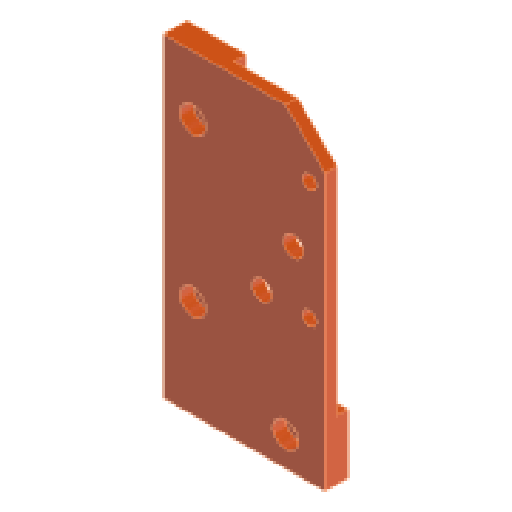
# Autodesk Inventor part: Alpha Idler Top
Saved by Autodesk Inventor 2023.2 (Build 272271000, 271)
## iProperties
Created: 2023-02-03
Part Number: Alpha Idler Top
Material: ABS Plastic
Document SubType Name: Modeling
Designer: remop
Density: 1.06 g/cm^3
Appearance: Smooth - Light Orange
Author: remop
Autodesk Inventor part; units mm, degrees
ref_plane "YZ Plane" through (0, 0, 0) normal (1, 0, 0) x (0, 1, 0)
ref_plane "XZ Plane" through (0, 0, 0) normal (0, 1, 0) x (-1, 0, 0)
ref_plane "XY Plane" through (0, 0, 0) normal (0, 0, 1) x (1, 0, 0)
sketch "Sketch1" plane through (0, 0, 0) normal (0, 0, 1) x (1, 0, 0)
  line L0 (-4, 11.7077) -> (6, 1.7077) projected
  line L1 (-4, 11.7077) -> (-5, 11.7077) projected
  arc A0 (-5, 11.7077) -> (-6, 10.7077) centre (-5, 10.7077) ccw projected
  line L2 (-6, 10.7077) -> (-6, -9.2784) projected
  arc A1 (-6, -9.2784) -> (-4.6842, -10.2272) centre (-5, -9.2784) ccw projected
  arc A2 (3.1184, -11.5061) -> (-4.6842, -10.2272) centre (-2, -18.2923) ccw projected
  arc A3 (3.1184, -11.5061) -> (3.7205, -11.7077) centre (3.7205, -10.7077) ccw projected
  line L3 (3.7205, -11.7077) -> (5, -11.7077) projected
  arc A4 (5, -11.7077) -> (6, -10.7077) centre (5, -10.7077) ccw projected
  line L4 (6, -10.7077) -> (6, 1.7077) projected
  arc A5 (5, -36.8923) -> (6, -35.8923) centre (5, -35.8923) ccw projected
  line L5 (6, -35.8923) -> (6, -27.7923) projected
  arc A6 (6, -27.7923) -> (5, -26.7923) centre (5, -27.7923) ccw projected
  line L6 (5, -26.7923) -> (-1.4303, -26.7923) projected
  arc A7 (-1.4303, -26.7923) -> (-2.3324, -28.2239) centre (-1.4303, -27.7923) ccw projected
  arc A8 (-2.2902, -35.4712) -> (-2.3324, -28.2239) centre (-10, -31.8923) ccw projected
  arc A9 (-2.2902, -35.4712) -> (-1.3832, -36.8923) centre (-1.3832, -35.8923) ccw projected
  line L7 (-1.3832, -36.8923) -> (5, -36.8923) projected
  line L8 (6, -53.1923) -> (6, -35.8923) projected
  line L9 (6, -27.7923) -> (6, -10.7077) projected
  line L10 (-5, 11.7077) -> (-20, 11.7077) projected
  line L11 (-20, 11.7077) -> (-35, 11.7077) projected
  line L12 (6, -68.1923) -> (6, -53.1923) projected
  line L13 (-35, 306.8077) -> (-35, -53.1923) projected
  line L14 (-35, -68.1923) -> (-35, -53.1923) projected
  line L15 (-20, -68.1923) -> (-35, -68.1923) projected
  line L16 (480, -68.1923) -> (-20, -68.1923) projected
  circle A10 centre (2, -2.1923) radius 1.4 projected
  circle A11 centre (2, -32.1923) radius 1.4 projected
  circle A12 centre (2, -2.1923) radius 1.75
  circle A13 centre (2, -32.1923) radius 1.75
  circle A14 centre (-10, -31.9923) radius 2.5 projected
  circle A15 centre (-2, -18.3923) radius 2.5 projected
  point P0 (0, 0)
  dimension "d18" = 3.5
  constraints: 2 centre point, 2 coincident, 1 equal radius
  measures "d18" diameter of A12
extrude "Extrusion1" add sketch "Sketch1" along normal blind 3 contours L0 L4 A4 L3 A3 A2 A1 L2 A0 L1 | A0 L2 A1 A2 A3 L3 A4 L9 A6 L6 A7 A8 A9 L7 A5 L8 L12 L16 L15 L14 L13 L11 L10 | L5 A5 L7 A9 A8 A7 L6 A6
sketch "Sketch2" plane through (0, 0, 0) normal (0, 0, -1) x (-1, 0, 0)
  line L0 (-6, -68.1923) -> (-6, 1.7077) projected
  line L1 (35, -68.1923) -> (-6, -68.1923) projected
  line L2 (35, 11.7077) -> (35, -68.1923) projected
  line L3 (4, 11.7077) -> (35, 11.7077) projected
  line L4 (-6, 1.7077) -> (4, 11.7077) projected
  line L5 (20, 11.7077) -> (20, -53.1923)
  line L6 (20, -53.1923) -> (-6, -53.1923)
  line L7 (-6, -68.1923) -> (-6, 1.7077) projected
  point P0 (0, 0)
  point P1 (7, -53.1923)
  dimension "d2" = 15
  dimension "d3" = 15
  constraints: 4 end point, 2 perpendicular, 2 point on line, 1 midpoint
  measures "d2" distance between parallel lines of L2 L5
  measures "d3" distance from line of L1 point (7, -53.192)
extrude "Extrusion2" add sketch "Sketch2" along normal blind 3 contours L0 L6 L5 L3 L2 L1
sketch "Sketch3" plane through (0, 0, 3) normal (0, 0, 1) x (1, 0, 0)
  line L0 (6, -68.1923) -> (6, 1.7077) projected
  line L1 (6, 1.7077) -> (-4, 11.7077) projected
  line L2 (-4, 11.7077) -> (-35, 11.7077) projected
  line L3 (-35, 11.7077) -> (-35, -68.1923) projected
  line L4 (-35, -68.1923) -> (6, -68.1923) projected
  circle A0 centre (2, -2.2923) radius 1.4 projected
  circle A1 centre (2, -32.2923) radius 1.4 projected
  point P0 (0, 0)
  point P1 (-27.5, -3.2923)
  point P2 (-27.5, -43.2923)
  point P3 (-4, -60.6923)
  dimension "d6" = 7.5
  dimension "d7" = 10
  dimension "d8" = 7.5
  dimension "d9" = 15
  dimension "d10" = 40
  constraints: 2 coincident, 1 vertical alignment
  measures "d6" distance from line of L4 point (-4, -60.692)
  measures "d7" distance from line of L0 point (-4, -60.692)
  measures "d8" distance from line of L3 point (-27.5, -43.292)
  measures "d9" distance from line of L2 point (-27.5, -3.292)
  measures "d10" distance of point (-27.5, -3.292) point (-27.5, -43.292)
hole "Hole1" at (-27.5, -3.2923, 3) at (-27.5, -43.2923, 3) at (-4, -60.6923, 3) direction (0, 0, -1) diameter 3.6 end through all counterbore diameter 6.5 counterbore depth 3.4 clearance for "Socket Head Cap Screw ISO 4762" size "M3" standard "ISO"
equation "\"d3\" = d2"
equation "\"d8\" = d6"
body "Solid1"
